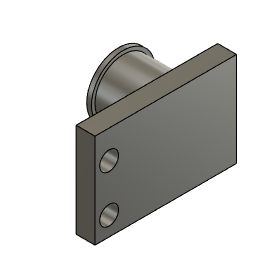
Крепление под ремни v7 (Autodesk Fusion 360 design; units mm, degrees)
Autodesk Fusion 360 part; units mm, degrees
sketch "Sketch1" plane through (0, 0, 0) normal (1, 0, 0) x (0, 0, -1)
  circle A0 centre (0, 0) radius 2
  line L0 (0.0008, 2) -> (0.0008, 8)
  line L1 (0.0008, 8) -> (0.0008, 10)
  circle A1 centre (0.0008, 10) radius 2
  line L2 (-3, 15) -> (27, 15)
  line L3 (27, 15) -> (27, -3)
  line L4 (27, -3) -> (-3, -3)
  line L5 (-3, -3) -> (-3, 15)
  circle A2 centre (18.0008, 7) radius 6
  circle A3 centre (18.0008, 7) radius 6.75
  dimension "d1" = 4
  dimension "d2" = 6
  dimension "d3" = 2
  dimension "d4" = 4
  dimension "d6" = 30
  dimension "d7" = 18
  dimension "d33" = 12
  dimension "d34" = 13.5
  dimension "d42" = 10
  dimension "d43" = 3
  constraint coincident A0.centre origin
  constraint coincident A0 L0.start
  constraint vertical L0
  constraint parallel L0 L1
  constraint coincident L1.end A1.centre
  constraint horizontal L2
  constraint vertical L3
  constraint horizontal L4
  constraint vertical L5
  constraint concentric A2 A3
  measures "d1" diameter of A0
  measures "d2" distance of L0.start L0.end
  measures "d3" distance of L0.end L1.end
  measures "d4" diameter of A1
  measures "d6" distance of L2.start L2.end
  measures "d7" distance of L2.start L4.end
  measures "d33" diameter of A2
  measures "d34" diameter of A3
  measures "d42" distance of L4 A2.centre
  measures "d43" distance of A0.centre L4
extrude "Extrude1" add sketch "Sketch1" along normal blind 4 contours L2 L3 L4 L5 | A2 | A3
extrude "Extrude2" add 1 faces at (1.3333, 15, -7) along direction (0, 1, 0) blind 1
extrude "Extrude3" add 1 faces at (1.3333, -3, -17) along direction (0, -1, 0) blind 1
extrude "Extrude8" add sketch "Sketch1" against normal blind 12 contours A2
extrude "Extrude9" add sketch "Sketch1" against normal blind 1 contours A3
sketch "Sketch5" plane through (-12, 0, 0) normal (-1, 0, 0) x (0, 0, 1)
  circle A0 centre (-18.0008, 7) radius 6
  circle A1 centre (-18.0008, 7) radius 6.75
  dimension "d39" = 13.5
  constraint concentric A0 A1
  measures "d39" diameter of A1
extrude "Extrude10" add sketch "Sketch5" against normal blind 1
